Autodesk Fusion 360 part; units mm, degrees
(part 2 of 2)
extrude "Extrude52" cut 1 faces at (-91.5, 87.9697, 10.4179) along direction (1, 0, 0) blind 15 on bodies 1 bodies 1
chamfer "Chamfer3" distance 10 angle 45 2 edges at (-71, 60, 28) (71, 60, 28) on bodies 1
chamfer "Chamfer4" distance 2 angle 45 41 edges at (-65.5, 60, 8) (-76.5, 60, 8) (-76.5, 65, 23) (-71, 60, 18) (-65.5, 65, 23) (-71, 70, 28) (-76.5, 82.5, 28) (-65.5, 79, 28) (-48.825, 95, 28) (48.825, 95, 28) (43.325, 88, 28) (-43.325, 88, 28) (76.5, 82.5, 28) (65.5, 79, 28) (65.5, 65, 23) (71, 70, 28) (76.5, 65, 23) (71, 60, 18) (65.5, 60, 8) (76.5, 60, 8) (76.5, 95, 9.675) (-76.5, 95, 9.675) (56.325, 95, 28) (0, -80, 28) (43.325, 88, 28) (0, -87, 28) (51.5, -83.5, 28) (-43.325, 88, 28) (0, -87, 28) (-51.5, -83.5, 28) (-56.325, 95, 28) (0, -80, 28) (51.5, -87, 13) (51.5, -80, 13) (-51.5, -80, 13) (-51.5, -87, 13) (-21.15, 112.7, 12.5) (21.15, 112.7, 12.5) (-21.15, 103.85, -8.65) (21.15, 103.85, -8.65) (0, 112.7, -8.65) 1 faces at (-7.05, 96.2333, 33.65) on bodies 1
sketch "Sketch44" plane through (0, 0, -2) normal (0, 0, 1) x (-1, 0, 0)
  line L0 (76.5, -62) -> (76.5, 87)
  line L1 (76.5, 87) -> (49.5, 87)
  line L2 (49.5, 87) -> (51.5, 85)
  line L3 (51.5, 85) -> (51.5, 82)
  line L4 (51.5, 82) -> (49.5, 80)
  line L5 (49.5, 80) -> (62.3, 80)
  line L6 (62.3, 80) -> (62.3, -88)
  line L7 (62.3, -88) -> (65.5, -88)
  line L8 (65.5, -88) -> (65.5, -62)
  line L9 (65.5, -62) -> (67.5, -60)
  line L10 (67.5, -60) -> (74.5, -60)
  line L11 (74.5, -60) -> (76.5, -62)
  circle A0 centre (-70, 80) radius 2.5
  dimension "d322" = 5
  measures "d322" diameter of A0
extrude "Extrude53" cut sketch "Sketch44" against normal blind 10 contours A0 bodies 1
pattern_linear "R-Pattern7" count 2 spacing 130 along (0, 1, 0) count 2 spacing 140 along (-1, 0, 0) of "Extrude53"
sketch "Sketch45" plane through (0, 88, 0) normal (0, -1, 0) x (1, 0, 0)
  line L0 (21.15, 31.65) -> (-21.15, 31.65)
  line L1 (-21.15, 31.65) -> (-21.15, 26)
  line L2 (-21.15, 26) -> (-65.5, 26)
  line L3 (-65.5, 26) -> (-65.5, -2)
  line L4 (-65.5, -2) -> (-62.3, -2)
  line L5 (-62.3, -2) -> (-59.3, -5)
  line L6 (-59.3, -5) -> (-59.3, -8.65)
  line L7 (-59.3, -8.65) -> (59.3, -8.65)
  line L8 (59.3, -8.65) -> (59.3, -5)
  line L9 (59.3, -5) -> (62.3, -2)
  line L10 (62.3, -2) -> (65.5, -2)
  line L11 (65.5, -2) -> (65.5, 26)
  line L12 (65.5, 26) -> (21.15, 26)
  line L13 (21.15, 26) -> (21.15, 31.65)
  circle A0 centre (15.5, -3) radius 1.6
  circle A1 centre (-15.5, -3) radius 1.6
  circle A2 centre (15.5, 28) radius 1.6
  circle A3 centre (-15.5, 28) radius 1.6
  circle A4 centre (40, 12.5) radius 4.5
  circle A5 centre (-40, 12.5) radius 4.5
  circle A6 centre (-15.5, 28) radius 3.5
  circle A7 centre (-15.5, -3) radius 3.5
  circle A8 centre (15.5, -3) radius 3.5
  circle A9 centre (15.5, 28) radius 3.5
  dimension "d329" = 7
  dimension "d330" = 7
  dimension "d331" = 7
  dimension "d332" = 7
  constraint concentric A3 A6
  constraint concentric A1 A7
  constraint concentric A0 A8
  constraint concentric A2 A9
  measures "d329" diameter of A6
  measures "d330" diameter of A7
  measures "d331" diameter of A8
  measures "d332" diameter of A9
extrude "Extrude54" cut sketch "Sketch45" against normal blind 15.7 contours A6 | A7 | A8 | A9 bodies 1
extrude "Extrude55" cut 1 faces at (-4.1667, 95, 8.3333) along direction (0, -1, 0) blind 7 on bodies 1 bodies 1
fillet "Fillet2" radius 6.5 4 edges at (-12.5, 100.35, 25) (-12.5, 100.35, 0) (12.5, 100.35, 25) (12.5, 100.35, 0) on bodies 1
sketch "Sketch46" plane through (0, 0, 0) normal (0, 0, 1) x (1, 0, 0)
  line L0 (-21, 88) -> (-21, 113)
  line L1 (-21, 113) -> (-80, 113)
  line L2 (-80, 113) -> (-80, -100)
  line L3 (-80, -100) -> (100, -100)
  line L4 (100, -100) -> (100, 100)
  line L5 (100, 100) -> (21.9148, 113)
  line L6 (21.9148, 113) -> (21.9148, 88.2807)
  line L7 (21.9148, 88.2807) -> (-21, 88)
  constraint vertical L0
  constraint perpendicular L0 L1
  constraint perpendicular L1 L2
  constraint perpendicular L2 L3
  constraint perpendicular L3 L4
  constraint parallel L4 L6
sketch "Sketch47" plane through (0, 95, 0) normal (0, 1, 0) x (-1, 0, 0)
  line L0 (-74.5, 26) -> (-74.5, -8.65)
  line L1 (-74.5, -8.65) -> (-19.15, -8.65)
  line L2 (-19.15, -8.65) -> (-21.15, -6.65)
  line L3 (-21.15, -6.65) -> (-21.15, 26)
  line L4 (-21.15, 26) -> (-74.5, 26)
  circle A0 centre (-40, 12.5) radius 4.5
  circle A1 centre (-40, 12.5) radius 6
  circle A2 centre (40, 12.5) radius 6
  dimension "d343" = 12
  dimension "d344" = 12
  constraint concentric A0 A1
  measures "d343" diameter of A1
  measures "d344" diameter of A2
extrude "Extrude58" add sketch "Sketch47" along normal blind 2 contours A0 | A1 | A2 bodies 1
fillet "Fillet3" radius 2 2 edges at (-34.406, 95, 14.6697) (45.594, 95, 14.6697) on bodies 1
sketch "Sketch48" plane through (0, 0, -2) normal (0, 0, 1) x (-1, 0, 0)
  circle A0 centre (-70, -50) radius 2.5
  circle A1 centre (-70, 80) radius 2.5
  line L0 (-76.5, 87) -> (-76.5, -62)
  line L1 (-76.5, -62) -> (-74.5, -60)
  line L2 (-74.5, -60) -> (-67.5, -60)
  line L3 (-67.5, -60) -> (-65.5, -62)
  line L4 (-65.5, -62) -> (-65.5, -88)
  line L5 (-65.5, -88) -> (-62.3, -88)
  line L6 (-62.3, -88) -> (-62.3, 80)
  line L7 (-62.3, 80) -> (-49.5, 80)
  line L8 (-49.5, 80) -> (-51.5, 82)
  line L9 (-51.5, 82) -> (-51.5, 85)
  line L10 (-51.5, 85) -> (-49.5, 87)
  line L11 (-49.5, 87) -> (-76.5, 87)
  line L12 (-56, 80) -> (-76.5, 80)
  line L13 (-76.5, 80) -> (-97.5, 80)
  line L14 (-97.5, 80) -> (-97.5, -11.8)
  line L15 (-56, 80) -> (-56, -11.8)
  line L16 (-56, -11.8) -> (-97.5, -11.8)
  line L17 (-97.5, -11.8) -> (-94.5, -11.8)
  line L18 (-94.5, -11.8) -> (-94.5, 80)
  line L19 (-94.5, 80) -> (-97.5, 80)
  line L20 (-97.5, 80) -> (-97.5, -11.8)
  dimension "d349" = 21
  dimension "d350" = 91.8
  dimension "d351" = 3
  constraint coincident L7 L12.start
  constraint coincident L0 L12.end
  constraint perpendicular L0 L12
  constraint perpendicular L0 L13
  constraint perpendicular L13 L14
  constraint perpendicular L7 L15
  constraint perpendicular L14 L16
  constraint horizontal L17
  constraint vertical L18
  constraint horizontal L19
  constraint vertical L20
  measures "d349" distance of L12.end L13.end
  measures "d350" distance of L13.end L14.end
  measures "d351" distance of L14.end L17.end
extrude "Extrude59" add sketch "Sketch48" along normal blind -6.65 and the other way blind -4 separate body contours A1 L0 L6 L12 L16 | A1 L12 | L6 L7 L12 L15 L16 | L0 L13 L16 L18 | L13 L14 L16 L17 L18 L19 L20 picked at (-69.6456, 78.4473) makes body 4
extrude "Extrude60" add sketch "Sketch48" along normal blind 21.35 contours L13 L14 L16 L17 L18 L19 L20 bodies 4
sketch "Sketch49" plane through (97.5, 0, 0) normal (1, 0, 0) x (0, 1, 0)
  line L0 (-80, 19.35) -> (-80, -8.65)
  line L1 (-80, -8.65) -> (11.8, -8.65)
  line L2 (11.8, -8.65) -> (11.8, 19.35)
  line L3 (11.8, 19.35) -> (-80, 19.35)
  line L4 (11.8, -8.65) -> (11.8, 12.35)
  line L5 (11.8, 12.35) -> (5.9, 12.35)
  circle A0 centre (5.9, 12.35) radius 1.75
  line L6 (5.9, 12.35) -> (-3.1, 12.35)
  line L7 (-3.1, 12.35) -> (-3.1, 15.35)
  line L8 (-3.1, 15.35) -> (-3.1, 9.35)
  line L9 (-3.1, 9.35) -> (-65.1, 9.35)
  line L10 (-65.1, 9.35) -> (-65.1, 15.35)
  line L11 (-65.1, 15.35) -> (-3.1, 15.35)
  line L12 (-65.1, 12.35) -> (-74.1, 12.35)
  circle A1 centre (-74.1, 12.35) radius 1.75
  dimension "d356" = 21
  dimension "d357" = 5.9
  dimension "d358" = 3.5
  dimension "d359" = 9
  dimension "d360" = 3
  dimension "d361" = 6
  dimension "d362" = 62
  dimension "d363" = 6
  dimension "d364" = 9
  dimension "d365" = 3.5
  constraint coincident L1.end L2.start
  constraint perpendicular L1 L4
  constraint perpendicular L4 L5
  constraint coincident L5.end A0.centre
  constraint perpendicular L2 L6
  constraint perpendicular L6 L7
  constraint perpendicular L6 L8
  constraint perpendicular L8 L9
  constraint perpendicular L9 L10
  constraint midpoint L10 L12.start
  constraint perpendicular L10 L12
  constraint coincident L12.end A1.centre
  measures "d356" distance of L1.end L4.end
  measures "d357" distance of L4.end L5.end
  measures "d358" diameter of A0
  measures "d359" distance of L5.end L6.end
  measures "d360" distance of L6.end L7.end
  measures "d361" distance of L7.end L8.end
  measures "d362" distance of L8.end L9.end
  measures "d363" distance of L9.end L10.end
  measures "d364" distance of L12.start L12.end
  measures "d365" diameter of A1
extrude "Extrude61" cut sketch "Sketch49" against normal blind 3 contours L5 A0 L6 | L5 A0 L6 | L7 L8 L9 L10 L11 | A1 bodies 4
combine "Combine1" operation cut target body 4 tool bodies 1
extrude "Extrude62" cut 1 faces at (70.4789, -78.4473, -8.65) along direction (0, 0, 1) blind 6.65 on bodies 4 bodies 4
hidden bodies 3
equation "d264 = 12.100 * 2 mm"
equation "d333 = -20.00 mm + 4.3 mm"

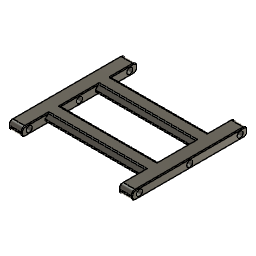
design "new outer arm"
Autodesk Fusion 360 part; units mm, degrees
sketch "Sketch1" plane through (0, 0, 0) normal (0, 0, 1) x (1, 0, 0)
  line L0 (0, 0) -> (0, 156)
  line L1 (0, 156) -> (18, 156)
  line L2 (18, 156) -> (18, 124.5)
  line L3 (18, 124.5) -> (149, 124.5)
  line L4 (149, 124.5) -> (149, 156)
  line L5 (149, 156) -> (167, 156)
  line L6 (167, 156) -> (167, 124.5)
  line L7 (167, 124.5) -> (167, 0)
  line L8 (167, 0) -> (149, 0)
  line L9 (149, 0) -> (149, 31.5)
  line L10 (149, 31.5) -> (18, 31.5)
  line L11 (18, 31.5) -> (18, 0)
  line L12 (18, 0) -> (0, 0)
  line L13 (18, 124.5) -> (18, 99.5)
  line L14 (18, 99.5) -> (149, 99.5)
  line L15 (149, 99.5) -> (149, 124.5)
  line L16 (18, 31.5) -> (18, 56.5)
  line L17 (18, 56.5) -> (149, 56.5)
  line L18 (149, 56.5) -> (149, 31.5)
  line L19 (18, 56.5) -> (18, 99.5)
  line L20 (149, 99.5) -> (149, 56.5)
  dimension "d1" = 156
  dimension "d2" = 18
  dimension "d3" = 31.5
  dimension "d4" = 131
  dimension "d5" = 18
  dimension "d6" = 31.5
  dimension "d7" = 131
  dimension "d8" = 25
  dimension "d9" = 25
  constraint coincident L0.start L12.end
  constraint vertical L0
  constraint perpendicular L0 L1
  constraint perpendicular L1 L2
  constraint perpendicular L2 L3
  constraint perpendicular L1 L4
  constraint perpendicular L4 L5
  constraint perpendicular L3 L6
  constraint perpendicular L3 L7
  constraint perpendicular L7 L8
  constraint perpendicular L8 L9
  constraint perpendicular L7 L10
  constraint perpendicular L8 L11
  constraint perpendicular L0 L12
  constraint perpendicular L3 L13
  constraint perpendicular L4 L14
  constraint perpendicular L3 L15
  constraint perpendicular L10 L16
  constraint perpendicular L9 L17
  constraint perpendicular L17 L18
  constraint perpendicular L14 L19
  measures "d1" distance of L0.start L0.end
  measures "d2" distance of L0.end L1.end
  measures "d3" distance of L1.end L2.end
  measures "d4" distance of L2.end L3.end
  measures "d5" distance of L4.end L5.end
  measures "d6" distance of L8.end L9.end
  measures "d7" distance of L9.end L10.end
  measures "d8" distance of L2.end L13.end
  measures "d9" distance of L10.end L16.end
extrude "Extrude1" add sketch "Sketch1" along normal blind 12 contours L0 L1 L2 L11 L12 L13 L16 L19 | L10 L16 L17 L18 | L3 L13 L14 L15 | L4 L5 L6 L7 L8 L9 L15 L18 L20
sketch "Sketch2" plane through (167, 0, 0) normal (1, 0, 0) x (0, 1, 0)
  line L0 (0, 0) -> (156, 0)
  line L1 (156, 0) -> (156, 12)
  line L2 (156, 12) -> (0, 12)
  line L3 (0, 12) -> (0, 0)
  line L4 (0, 6) -> (10, 6)
  circle A0 centre (10, 6) radius 4
  line L5 (10, 6) -> (78, 6)
  circle A1 centre (78, 6) radius 4
  line L6 (156, 6) -> (146, 6)
  circle A2 centre (146, 6) radius 4
  dimension "d12" = 10
  dimension "d13" = 8
  dimension "d14" = 68
  dimension "d15" = 8
  dimension "d16" = 10
  dimension "d17" = 8
  constraint midpoint L3 L4.start
  constraint perpendicular L3 L4
  constraint coincident L4.end A0.centre
  constraint parallel L4 L5
  constraint coincident L5.end A1.centre
  constraint midpoint L1 L6.start
  constraint perpendicular L1 L6
  constraint coincident L6.end A2.centre
  measures "d12" distance of L4.start L4.end
  measures "d13" diameter of A0
  measures "d14" distance of L4.end L5.end
  measures "d15" diameter of A1
  measures "d16" distance of L6.start L6.end
  measures "d17" diameter of A2
extrude "Extrude2" cut sketch "Sketch2" against normal blind 167 contours L4 A0 L5 | L4 A0 L5 | A1 | A2
fillet "Fillet1" radius 5 8 edges at (158, 0, 12) (9, 0, 12) (9, 0, 0) (158, 156, 12) (158, 156, 0) (9, 156, 12) (9, 156, 0) (158, 0, 0)
chamfer "Chamfer2" distance 5 angle 45 8 edges at (83.5, 31.5, 12) (83.5, 56.5, 12) (83.5, 56.5, 0) (83.5, 31.5, 0) (83.5, 99.5, 0) (83.5, 99.5, 12) (83.5, 124.5, 0) (83.5, 124.5, 12)
chamfer "Chamfer1" distance 1 angle 45 14 faces at (161, 69.1667, 12) (6, 152.8583, 11.6418) (6, 156, 6.3333) (6, 152.6353, 0.275) (161, 69.1667, 0) (161, 0.0057, 4.7621) (161, 0, 5.6667) (161, 0.0226, 7.4753) (12, 4.5247, 0.0226) (12, 0, 5.6667) (12, 4.5247, 11.9774) (155, 152.6353, 0.275) (155, 156, 5.6667) (155, 152.6353, 11.725)

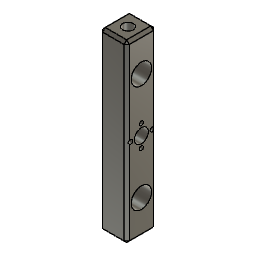
design "slider"
Autodesk Fusion 360 part; units mm, degrees
sketch "Sketch1" plane through (0, 0, 0) normal (0, 0, 1) x (1, 0, 0)
  line L0 (10, -11) -> (-10, -11)
  line L1 (-10, -11) -> (-10, 11)
  line L2 (-10, 11) -> (10, 11)
  line L3 (10, 11) -> (10, -11)
  line L4 (10, -11) -> (-10, 11) construction
  line L5 (-10, -11) -> (10, 11) construction
  circle A0 centre (0, 0) radius 4
  dimension "d1" = 20
  dimension "d2" = 22
  dimension "d75" = 8
  constraint horizontal L0
  constraint perpendicular L0 L1
  constraint parallel L0 L2
  constraint parallel L1 L3
  measures "d1" distance of L1.end L2.end
  measures "d2" distance of L0.end L1.end
  measures "d75" diameter of A0
extrude "Extrude1" add sketch "Sketch1" along normal blind 131 contours L0 L1 L2 L3 | A0
sketch "Sketch3" plane through (0, 0, 131) normal (0, 0, 1) x (-1, 0, 0)
  line L0 (-10, -11) -> (10, -11)
  line L1 (10, -11) -> (10, 11)
  line L2 (10, 11) -> (-10, 11)
  line L3 (-10, 11) -> (-10, -11)
  circle A0 centre (0, 0) radius 4
  dimension "d21" = 8
  measures "d21" diameter of A0
extrude "Extrude5" cut sketch "Sketch3" against normal blind 10 contours A0
extrude "Extrude6" cut sketch "Sketch1" along normal blind 10 contours A0
sketch "Sketch5" plane through (10, 0, 0) normal (1, 0, 0) x (0, 1, 0)
  line L0 (-11, 0) -> (11, 0)
  line L1 (11, 0) -> (11, 131)
  line L2 (-11, 131) -> (-11, 0)
  circle A0 centre (0, 65.5) radius 5.2
  line L3 (0, 65.5) -> (0, 25.5)
  circle A1 centre (0, 25.5) radius 7.6
  line L4 (0, 65.5) -> (0, 105.5)
  circle A2 centre (0, 105.5) radius 7.6
  line L5 (11, 131) -> (-11, 131)
  dimension "d40" = 40
  dimension "d41" = 15.2
  dimension "d42" = 40
  dimension "d43" = 15.2
  dimension "d60" = 10.4
  constraint coincident A0.centre L3.start
  constraint vertical L3
  constraint coincident L3.end A1.centre
  constraint parallel L3 L4
  constraint coincident L4.end A2.centre
  measures "d40" distance of A0.centre L3.end
  measures "d41" diameter of A1
  measures "d42" distance of A0.centre L4.end
  measures "d43" diameter of A2
  measures "d60" diameter of A0
extrude "Extrude8" cut sketch "Sketch5" against normal blind 20 contours A0 L3 L4 | A0 L3 L4 | A1 | A2
sketch "Sketch6" plane through (-10, 0, 0) normal (-1, 0, 0) x (0, -1, 0)
  circle A0 centre (0, 105.5) radius 7.6
  circle A1 centre (0, 25.5) radius 7.6
  line L0 (-11, 0) -> (11, 0)
  line L1 (11, 0) -> (11, 131)
  line L2 (-11, 131) -> (-11, 0)
  circle A2 centre (0, 25.5) radius 9
  circle A3 centre (0, 105.5) radius 9
  circle A4 centre (0, 105.5) radius 4.2
  circle A5 centre (0, 25.5) radius 4.2
  circle A6 centre (0, 65.5) radius 5.2
  line L3 (11, 131) -> (-11, 131)
  dimension "d48" = 18
  dimension "d49" = 18
  dimension "d54" = 8.4
  dimension "d55" = 8.4
  constraint concentric A1 A2
  constraint concentric A0 A3
  constraint concentric A3 A4
  constraint concentric A1 A5
  measures "d48" diameter of A2
  measures "d49" diameter of A3
  measures "d54" diameter of A4
  measures "d55" diameter of A5
extrude "Extrude10" add sketch "Sketch6" against normal blind 2 contours A0 | A1 | A2 | A3
sketch "Sketch10" plane through (10, 0, 0) normal (1, 0, 0) x (0, 1, 0)
  circle A0 centre (0, 105.5) radius 7.6
  circle A1 centre (0, 25.5) radius 7.6
  circle A2 centre (0, 65.5) radius 5.2
  line L0 (-11, 0) -> (11, 0)
  line L1 (11, 0) -> (11, 131)
  line L2 (-11, 131) -> (-11, 0)
  line L3 (0, 65.5) -> (8, 65.5)
  circle A3 centre (8, 65.5) radius 1.5
  line L4 (11, 131) -> (-11, 131)
  dimension "d67" = 8
  dimension "d68" = 3
  constraint coincident A2.centre L3.start
  constraint horizontal L3
  constraint coincident L3.end A3.centre
  measures "d67" distance of A2.centre L3.end
  measures "d68" diameter of A3
extrude "Extrude13" cut sketch "Sketch10" against normal blind 20 contours A3
pattern_circular "C-Pattern2" count 4 over 360 about axis through (10, 0, 65.5) along (-1, 0, 0) of "Extrude13"
chamfer "Chamfer1" distance 2 angle 45 8 edges at (0, 11, 0) (10, 0, 0) (-10, 0, 0) (0, -11, 0) (-10, 0, 131) (0, -11, 131) (10, 0, 131) (0, 11, 131) 2 faces at (3.3333, -11, 43.6667) (-3.3333, 11, 43.6667)
equation "d6 = 161 mm - 30 mm"
